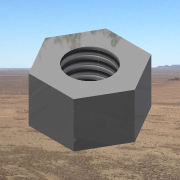
# Autodesk Inventor part: 0nut_ss_375
Saved by Autodesk Inventor 2013 SP2 (Build 170200200, 200)
## iProperties
Company: HERA Project
Created: 2013-07-11
Part Number: 0nut_ss_375
Material: Stainless Steel
Document SubType Name: Modeling
Designer: Dave
Density: 8.08 g/cm^3
Mass: 8.68893 g
Surface Area: 8.74722 cm^2
Volume: 1.07536 cm^3
Description: 0.375 stainless  nut
Author: David DeBoer
Autodesk Inventor part; units mm, degrees
ref_plane "YZ Plane" through (0, 0, 0) normal (1, 0, 0) x (0, 1, 0)
ref_plane "XZ Plane" through (0, 0, 0) normal (0, 1, 0) x (-1, 0, 0)
ref_plane "XY Plane" through (0, 0, 0) normal (0, 0, 1) x (1, 0, 0)
sketch "Sketch1" plane through (0, 0, 0) normal (0, 1, 0) x (-1, 0, 0)
  line L0 (8.2489, 0) -> (4.1244, -7.1437)
  line L1 (4.1244, -7.1437) -> (-4.1244, -7.1437)
  line L2 (-4.1244, -7.1437) -> (-8.2489, 0)
  line L3 (-8.2489, 0) -> (-4.1244, 7.1437)
  line L4 (-4.1244, 7.1437) -> (4.1244, 7.1437)
  line L5 (4.1244, 7.1437) -> (8.2489, 0)
  point P0 (0, 0)
  point P1 (0, 0)
  dimension "d0" = 14.2875
  constraints: 12 end point, 1 coincident, 13 other
  measures "d0" distance between parallel lines of L1 L4
extrude "Extrusion1" add sketch "Sketch1" along normal blind 8.3344
sketch "Sketch2" plane through (0, 8.3344, 0) normal (0, 1, 0) x (1, 0, 0)
  circle A0 centre (0, 0) radius 4.7625
  dimension "d3" = 9.525
  constraints: 1 centre point, 1 coincident
  measures "d3" diameter of A0
hole "Hole1" at (0, 8.3344, 0) direction (0, -1, 0) diameter 7.7978 end through all thread size "3/8-16 UNC" class "2B" standard "ANSI Unified Screw Threads"
body "Solid1"
